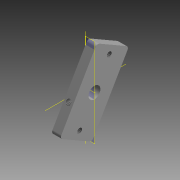
# Autodesk Inventor part: spring_arm
Saved by Autodesk Inventor 2015 (Build 190159000, 159)
## iProperties
Created: 2015-09-03
Part Number: spring_arm
Material: Generic
Description: insert part description/title
Document SubType Name: Modeling
Designer: francis
Density: 1 g/cm^3
Appearance: Default
Part Category: insert part category here and press enter to fill value
Author: francis
Autodesk Inventor part; units mm, degrees
ref_plane "YZ Plane" through (0, 0, 0) normal (1, 0, 0) x (0, 1, 0)
ref_plane "XY Plane" through (0, 0, 0) normal (0, 0, 1) x (1, 0, 0)
sketch "Sketch1" plane through (0, 0, 0) normal (1, 0, 0) x (0, 1, 0)
  line L0 (4.3253, -17.5083) -> (17.3253, 5.0083)
  line L1 (12.933, 21.4006) -> (12.067, 21.9006)
  line L2 (-4.3253, 17.5083) -> (-17.3253, -5.0083)
  line L3 (-12.933, -21.4006) -> (-12.067, -21.9006)
  line L4 (10.8253, -6.25) -> (-10.8253, 6.25) construction
  arc A0 (17.3253, 5.0083) -> (12.933, 21.4006) centre (6.933, 11.0083) ccw
  arc A1 (12.067, 21.9006) -> (-4.3253, 17.5083) centre (6.067, 11.5083) ccw
  arc A2 (-17.3253, -5.0083) -> (-12.933, -21.4006) centre (-6.933, -11.0083) ccw
  arc A3 (-12.067, -21.9006) -> (4.3253, -17.5083) centre (-6.067, -11.5083) ccw
  line L5 (-29.5294, 0) -> (32.1344, 0) construction
  line L6 (0, -39.0609) -> (0, 39.0609) construction
  point P0 (0, 0)
  point P1 (-1.6747, -27.9006)
  point P2 (23.3253, 15.4006)
  point P3 (1.6747, 27.9006)
  dimension "d1" = 25
  dimension "d2" = 50
  dimension "d3" = 12
  dimension "d4" = 60
  constraints: 10 end point, 8 point on circle, 8 tangent, 6 point on line, 4 centre point, 3 equal radius, 3 midpoint, 3 perpendicular
  measures "d1" distance of point (23.325, 15.401) point (1.675, 27.901)
  measures "d2" distance of point (-1.675, -27.901) point (23.325, 15.401)
  measures "d3" radius of A0
  measures "d4" angle of L5 L2
extrude "Extrusion1" add sketch "Sketch1" along normal blind 6
sketch "Sketch2" plane through (0, 0, 0) normal (-1, 0, 0) x (0, 0, 1)
  point P0 (0, 0)
hole "Hole1" at (0, 0, 0) direction (1, 0, 0) diameter 8 end through all
sketch "Sketch3" plane through (0, 0, 0) normal (0, 1, 0) x (-1, 0, 0)
  line L0 (-6, -17.5083) -> (-6, 5.0083) construction
  line L1 (0, 5.0083) -> (0, -17.5083) construction
  line L2 (1.2, 0) -> (-7.2, 0) construction
  line L3 (0, 0) -> (-6, 0) construction
  point P0 (-3, 0)
  point P1 (-3, 0)
  constraints: 2 end point, 2 point on line, 1 coincident, 1 midpoint
hole "Hole2" at (3, 0, 0) at (3, 0, 0) direction (0, -1, 0) diameter 3.242 end through all thread size "M4x0.7" class "6H" standard "ISO Metric profile"
sketch "Sketch4" plane through (0, 0, 0) normal (-1, 0, 0) x (0, 0, 1)
  circle A0 centre (0, 0) radius 4 construction
  line L0 (5.0083, 17.3253) -> (-17.5083, 4.3253) construction
  arc A1 (-17.5083, 4.3253) -> (-21.9006, -12.067) centre (-11.5083, -6.067) ccw construction
  line L1 (-21.9006, -12.067) -> (-21.4006, -12.933) construction
  arc A2 (-21.4006, -12.933) -> (-5.0083, -17.3253) centre (-11.0083, -6.933) ccw construction
  line L2 (-5.0083, -17.3253) -> (17.5083, -4.3253) construction
  arc A3 (17.5083, -4.3253) -> (21.9006, 12.067) centre (11.5083, 6.067) ccw construction
  line L3 (21.9006, 12.067) -> (21.4006, 12.933) construction
  arc A4 (21.4006, 12.933) -> (5.0083, 17.3253) centre (11.0083, 6.933) ccw construction
  line L4 (-26.825, -15.4874) -> (32.6029, 18.8233) construction
  line L5 (5.0083, 17.3253) -> (-17.5083, 4.3253) construction
  point P0 (17.3205, 10)
  point P1 (-17.3205, -10)
  dimension "d21" = 20
  dimension "d22" = 20
  constraints: 3 point on line, 2 end point, 1 parallel
  measures "d21" distance of point (0, 0) point (17.321, 10)
  measures "d22" distance of point (0, 0) point (-17.321, -10)
hole "Hole3" at (0, 10, 17.3205) at (0, -10, -17.3205) direction (1, 0, 0) diameter 3.242 end through all thread size "M4x0.7" class "6H" standard "ISO Metric profile"
body "Solid1"
